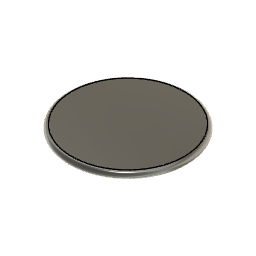
Back_Part v1 (Autodesk Fusion 360 design; units mm, degrees)
Autodesk Fusion 360 part; units mm, degrees
sketch "Esquisse1" plane through (0, 0, 0) normal (0, 0, 1) x (1, 0, 0)
  circle A0 centre (0, 0) radius 37.5
  dimension "d1" = 75
  constraint coincident A0.centre origin
  measures "d1" diameter of A0
extrude "Extrusion1" add sketch "Esquisse1" along normal blind 4
sketch "Esquisse2" plane through (0, 0, 0) normal (0, 0, 1) x (1, 0, 0)
  line L0 (50, 50) -> (-50, 50)
  line L1 (-50, 50) -> (-50, -50)
  line L2 (-50, -50) -> (50, -50)
  line L3 (50, -50) -> (50, 50)
  line L4 (0, 50) -> (0, -50)
  line L5 (50, 0) -> (-50, 0)
  line L6 (-50, 50) -> (50, -50)
  line L7 (50, 50) -> (-50, -50)
  line L8 (50, -20) -> (-50, -20)
  line L9 (50, 20) -> (-50, 20)
  constraint horizontal L0
  constraint vertical L1
  constraint horizontal L2
  constraint vertical L3
  constraint midpoint L0 L4.start
  constraint midpoint L2 L4.end
  constraint midpoint L3 L5.start
  constraint midpoint L1 L5.end
  constraint perpendicular L6 L7
  constraint coincident L3 L8.start
  constraint coincident L1 L8.end
  constraint perpendicular L1 L8
  constraint coincident L3 L9.start
  constraint coincident L1 L9.end
  constraint perpendicular L1 L9
hole "Perçage1" at (-0.2221, -19.9867, 0) direction (0, 0, 1) diameter 6 depth 2 tip angle 180
hole "Perçage2" at (-19.3001, 20.092, 0) direction (0, 0, 1) diameter 6 depth 2 tip angle 180
hole "Perçage3" at (19.5955, 19.9441, 0) direction (0, 0, 1) diameter 6 depth 2 tip angle 180
fillet "Congé1" radius 5 1 faces at (9.3028, 10.3652, 4)
fillet "Congé2" radius 2 1 edges at (-34.9623, -13.5606, 0)
